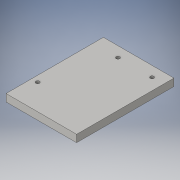
# Autodesk Inventor part: Base
Saved by Autodesk Inventor 2016 (Build 200138000, 138)
## iProperties
Created: 2018-09-18
Part Number: Base
Material: Generic
Document SubType Name: Modeling
Designer: Kyle
Density: 1 g/cm^3
Appearance: Default
Author: Kyle
Autodesk Inventor part; units mm, degrees
ref_plane "YZ Plane" through (0, 0, 0) normal (1, 0, 0) x (0, 1, 0)
ref_plane "XZ Plane" through (0, 0, 0) normal (0, 1, 0) x (-1, 0, 0)
ref_plane "XY Plane" through (0, 0, 0) normal (0, 0, 1) x (1, 0, 0)
sketch "Sketch1" plane through (0, 0, 0) normal (0, 1, 0) x (-1, 0, 0)
  line L0 (-29, 40) -> (29, 40)
  line L1 (29, 40) -> (29, -40)
  line L2 (29, -40) -> (-29, -40)
  line L3 (-29, -40) -> (-29, 40)
  line L4 (-29, 40) -> (29, -40) construction
  line L5 (29, 40) -> (-29, -40) construction
  line L6 (29, 40) -> (29, 13)
  line L7 (-29, -40) -> (-17, -40)
  line L8 (-29, -40) -> (11, -40)
  circle A0 centre (8.5, -31.5) radius 1.5
  circle A1 centre (-19.5, -31.5) radius 1.5
  circle A2 centre (-19.5, -31.5) radius 1.5
  circle A3 centre (24, 19) radius 1.5
  line L9 (0, 0) -> (0, 17.5)
  line L10 (0, 17.5) -> (0, 19)
  line L11 (0, 19) -> (24, 19)
  line L12 (0, 0) -> (0, -31.5)
  line L13 (0, -31.5) -> (8.5, -31.5)
  line L14 (0, -31.5) -> (-19.5, -31.5)
  dimension "d0" = 58
  dimension "d1" = 80
  dimension "d5" = 3
  dimension "d6" = 3
  dimension "d7" = 3
  dimension "d10" = 17.5
  dimension "d11" = 8.5
  dimension "d12" = 19.5
  dimension "d13" = 31.5
  dimension "d14" = 24
  constraints: 30 end point, 5 point on line, 4 centre point, 4 perpendicular, 3 horizontal, 2 midpoint, 2 parallel, 2 vertical, 1 coincident, 1 concentric
  measures "d0" distance of L1.end L3.start
  measures "d1" distance of L1.start L1.end
  measures "d5" diameter of A0
  measures "d6" diameter of A1
  measures "d7" diameter of A3
  measures "d10" distance of L9.start L9.end
  measures "d11" distance of L12.end L13.end
  measures "d12" distance of L12.end L14.end
  measures "d13" distance of L9.start L12.end
  measures "d14" distance of L10.end L11.end
extrude "Extrusion1" add sketch "Sketch1" along normal blind 6
body "Solid1"
